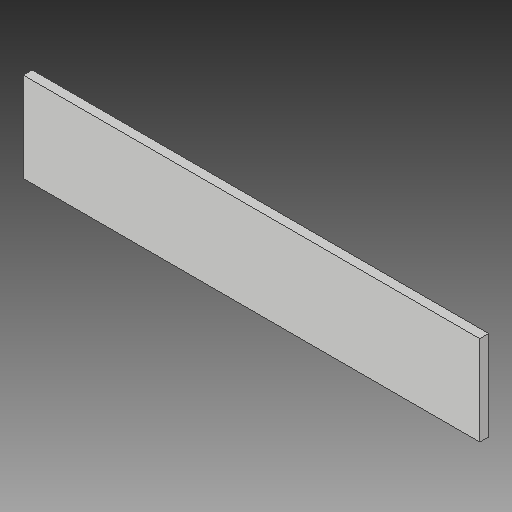
# Autodesk Inventor part: Frame bottom Left
Saved by Autodesk Inventor 2019 (Build 230136000, 136)
## iProperties
Created: 2018-10-20
Part Number: Frame bottom Left
Material: Generic
Document SubType Name: Modeling
Designer: LillaHunden
Density: 1 g/cm^3
Appearance: Default
Mass: 63.75 g
Surface Area: 285.5 cm^2
Volume: 63.75 cm^3
Author: LillaHunden
Autodesk Inventor part; units mm, degrees
ref_plane "YZ Plane" through (0, 0, 0) normal (1, 0, 0) x (0, 1, 0)
ref_plane "XZ Plane" through (0, 0, 0) normal (0, 1, 0) x (-1, 0, 0)
ref_plane "XY Plane" through (0, 0, 0) normal (0, 0, 1) x (1, 0, 0)
sketch "Sketch1" plane through (0, 0, 0) normal (0, 0, 1) x (1, 0, 0)
  line L0 (0, 0) -> (270, 0) construction
  line L1 (270, 0) -> (270, 10) construction
  line L2 (0, 10) -> (270, 10) construction
  line L3 (0, 0) -> (0, 10) construction
  line L4 (0, 50) -> (0, 0) construction
  line L5 (0, 50) -> (-5, 50) construction
  line L6 (-5, 0) -> (-5, 50) construction
  line L7 (0, 0) -> (-5, 0) construction
  line L8 (-5, 0) -> (250, 0)
  line L9 (250, 0) -> (250, 50)
  line L10 (250, 50) -> (-5, 50)
  line L11 (-5, 50) -> (-5, 0)
  constraints: 8 end point, 2 parallel, 1 horizontal, 1 perpendicular
extrude "Extrusion1" add sketch "Sketch1" along normal blind 5
body "Solid1"
